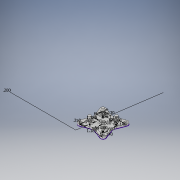
# Autodesk Inventor part: Gryo Mount
Saved by Autodesk Inventor 2017 (Build 210142000, 142)
## iProperties
Created: 2017-05-14
Part Number: Gryo Mount
Material: Generic
Document SubType Name: Modeling
Designer: Eric the Great
Density: 1 g/cm^3
Appearance: Default
Author: Eric the Great
Autodesk Inventor part; units mm, degrees
ref_plane "YZ Plane" through (0, 0, 0) normal (1, 0, 0) x (0, 1, 0)
ref_plane "XZ Plane" through (0, 0, 0) normal (0, 1, 0) x (-1, 0, 0)
ref_plane "XY Plane" through (0, 0, 0) normal (0, 0, 1) x (1, 0, 0)
sketch "Sketch1" plane through (0, 0, 0) normal (0, 1, 0) x (-1, 0, 0)
  line L0 (-8.95, 8.85) -> (-8.95, -8.85)
  line L1 (-8.95, -8.85) -> (8.95, -8.85)
  line L2 (8.95, -8.85) -> (8.95, 8.85)
  line L3 (8.95, 8.85) -> (-8.95, 8.85)
  line L4 (-8.95, 8.85) -> (8.95, -8.85) construction
  line L5 (-8.95, -8.85) -> (8.95, 8.85) construction
  circle A0 centre (8.95, 8.85) radius 1.775
  circle A1 centre (8.95, -8.85) radius 1.775
  circle A2 centre (-8.95, 8.85) radius 1.775
  circle A3 centre (-8.95, -8.85) radius 1.775
  circle A4 centre (8.95, 8.85) radius 2.54
  circle A5 centre (8.95, -8.85) radius 2.54
  circle A6 centre (-8.95, 8.85) radius 2.54
  circle A7 centre (-8.95, -8.85) radius 2.54
  line L6 (2.2577, 2.2325) -> (2.2451, 2.2451)
  circle A8 centre (15.1, -15.1) radius 1.65
  circle A9 centre (15.1, 15.1) radius 1.65
  circle A10 centre (-15.1, -15.1) radius 1.65
  circle A11 centre (-15.1, 15.1) radius 1.65
  line L7 (0, 0) -> (4.4901, 0)
  line L8 (0, 0) -> (0, 3.0635)
  line L9 (-15.1, 15.1) -> (15.1, -15.1) construction
  circle A12 centre (15.1, 15.1) radius 3.175
  circle A13 centre (15.1, -15.1) radius 3.175
  circle A14 centre (-15.1, 15.1) radius 3.175
  circle A15 centre (-15.1, -15.1) radius 3.175
  line L10 (18.0638, 13.9613) -> (12.7, 0)
  line L11 (12.7, 0) -> (18.0638, -13.9613)
  line L12 (13.9613, 18.0638) -> (0, 12.7)
  line L13 (0, 12.7) -> (-13.9613, 18.0638)
  line L14 (-18.0638, 13.9613) -> (-12.7, 0)
  line L15 (-12.7, 0) -> (-18.0638, -13.9613)
  line L16 (-13.9613, -18.0638) -> (0, -12.7)
  line L17 (0, -12.7) -> (13.9613, -18.0638)
  point P0 (0, -0.2784)
  point P1 (-0.5887, -0.5887)
  point P2 (-4.5282, -4.9254)
  point P3 (0, 0)
  dimension "d0" = 17.7
  dimension "d1" = 17.9
  dimension "d2" = 3.55
  dimension "d3" = 3.55
  dimension "d4" = 3.55
  dimension "d5" = 3.55
  dimension "d11" = 5.08
  dimension "d12" = 5.08
  dimension "d13" = 5.08
  dimension "d14" = 5.08
  dimension "d31" = 3.3
  dimension "d34" = 30.2
  dimension "d37" = 30.2
  dimension "d68" = 6.35
  dimension "d71" = 30.2
  dimension "d74" = 30.2
  dimension "d78" = 12.7
  dimension "d79" = 12.7
  dimension "d81" = 12.7
  constraints: 38 end point, 16 centre point, 9 coincident, 8 point on circle, 8 tangent, 7 midpoint, 4 point on line, 4 vertical, 3 horizontal, 3 perpendicular, 2 parallel, 15 other
  measures "d0" distance of L0.start L0.end
  measures "d1" distance of L1.end L0.end
  measures "d2" diameter of A0
  measures "d3" diameter of A1
  measures "d4" diameter of A2
  measures "d5" diameter of A3
  measures "d11" diameter of A4
  measures "d12" diameter of A5
  measures "d13" diameter of A6
  measures "d14" diameter of A7
  measures "d31" diameter of A8
  measures "d34" distance of L9.end A9.centre
  measures "d37" distance of L9.end A10.centre
  measures "d68" diameter of A12
  measures "d71" distance of A12.centre A13.centre
  measures "d74" distance of A12.centre A14.centre
  measures "d78" distance of point (0, 0) L10.end
  measures "d79" distance of point (0, 0) L16.end
  measures "d81" distance of L12.end point (0, 0)
extrude "Extrusion2" add sketch "Sketch1" along normal blind 10 contours L3 A2 L0 | L0 A2 L3 | A3 L1 L0 | L0 L1 A3 | A0 L2 L3 | L3 L2 A0 | A1 L2 L1 | L1 L2 A1
extrude "Extrusion3" add sketch "Sketch1" along normal blind 6 contours A2 L3 A6 L0 | L0 A6 L3 A2 | A7 L1 A3 L0 | L0 A3 L1 A7 | A4 L2 A0 L3 | L3 A0 L2 A4 | A5 L2 A1 L1 | L1 A1 L2 A5
extrude "Extrusion6" add sketch "Sketch1" along normal blind 2.5 contours L3 A2 L0 | A2 L3 A6 L0 | A6 L3 A4 L2 A5 L1 A7 L0 | A7 L1 A3 L0 | L3 A0 L2 A4 | A3 L1 L0 | L3 L2 A0 | A5 L2 A1 L1 | A1 L2 L1 | A12 | A12 L10 L11 A13 L17 L16 A15 L15 L14 A14 L13 L12 | A14 | A13 | A15 picked at (-7.7815, 8.7183) picked at (-6.6862, 8.6616) picked at (-6.6862, -8.6616) picked at (6.7011, 8.5299) picked at (-8.5616, -7.7401) picked at (7.7815, 8.7183) picked at (6.8287, -8.0375) picked at (8.8183, -7.6815)
fillet "Fillet2" radius 10 4 edges at (0, 1.25, 12.7) (12.7, 1.25, 0) (0, 1.25, -12.7) (-12.7, 1.25, 0)
fillet "Fillet3" radius 2 4 edges at (-6.41, 2.5, 8.85) (11.49, 2.5, 8.85) (11.49, 2.5, -8.85) (-6.41, 2.5, -8.85)
equation "\"d3\" = d2"
equation "\"d4\" = d2"
equation "\"d5\" = d2"
equation "\"d12\" = d11"
equation "\"d13\" = d11"
equation "\"d14\" = d11"
body "Solid1"
